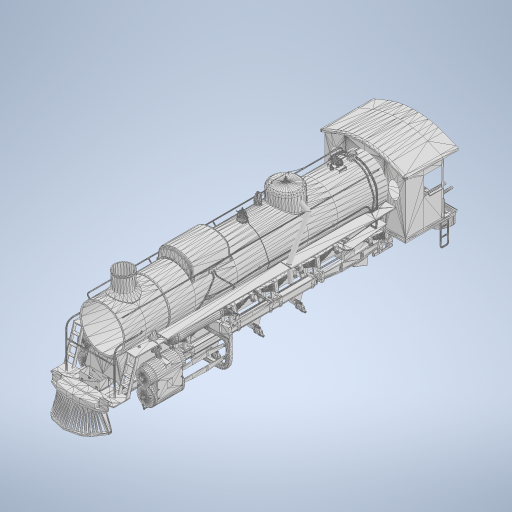
# Autodesk Inventor part: dry_pipe
Saved by Autodesk Inventor 2023 (Build 270158000, 158)
## iProperties
Created: 2023-09-04
Part Number: dry_pipe
Material: Generic
Document SubType Name: Modeling
Designer: Peter
Density: 1 g/cm^3
Appearance: Default
Author: Peter
Autodesk Inventor part; units mm, degrees
ref_plane "YZ Plane" through (0, 0, 0) normal (1, 0, 0) x (0, 1, 0)
ref_plane "XZ Plane" through (0, 0, 0) normal (0, 1, 0) x (-1, 0, 0)
ref_plane "XY Plane" through (0, 0, 0) normal (0, 0, 1) x (1, 0, 0)
ref_plane "Work Plane1" through (280.9318, 3704.4454, -1110.6402) normal (0.8456, -0.5338, 0.0033) x (0.5338, 0.8456, 0)
sketch "Sketch1" plane through (280.9318, 3704.4454, -1110.6402) normal (0.8456, -0.5338, 0.0033) x (0.5338, 0.8456, 0)
  circle A0 centre (0, 0) radius 76.2
  point P0 (-3282.5371, 1104.8673)
  dimension "d2" = 152.4
  constraints: 1 centre point
  measures "d2" diameter of A0
sketch3d "3D Sketch1"
  line L0 (280.9318, 3704.4454, -1110.6402) -> (825.914, 3360.445, -1108.5039)
  line L1 (825.914, 3360.445, -1108.5039) -> (1026.3105, 2255.7781, -198.6163)
  line L2 (1026.3105, 2255.7781, -198.6163) -> (1105.9021, 1687.4369, -184.3233)
sweep "Sweep1" add profiles "Sketch1" path "3D Sketch1"
body "Solid1"
